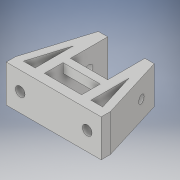
# Autodesk Inventor part: GT2_Holder
Saved by Autodesk Inventor 2018 (Build 220112000, 112)
## iProperties
Created: 2017-10-14
Part Number: GT2_Holder
Material: Generic
Document SubType Name: Modeling
Designer: Jurjen
Density: 1 g/cm^3
Appearance: Default
Author: Jurjen
Autodesk Inventor part; units mm, degrees
ref_plane "YZ Plane" through (0, 0, 0) normal (1, 0, 0) x (0, 1, 0)
ref_plane "XZ Plane" through (0, 0, 0) normal (0, 1, 0) x (-1, 0, 0)
ref_plane "XY Plane" through (0, 0, 0) normal (0, 0, 1) x (1, 0, 0)
sketch "Sketch1" plane through (0, 0, 0) normal (0, 0, 1) x (1, 0, 0)
  line L0 (-25.5, 10) -> (25.5, 10)
  line L1 (25.5, 10) -> (25.5, -10)
  line L2 (25.5, -10) -> (-25.5, -10)
  line L3 (-25.5, -10) -> (-25.5, 10)
  point P0 (0, 0)
  point P1 (0, 10)
  point P2 (25.5, 0)
  dimension "d0" = 51
  dimension "d1" = 20
  constraints: 8 end point, 2 midpoint, 2 parallel, 1 horizontal, 1 horizontal alignment, 1 perpendicular, 1 vertical alignment
  measures "d0" distance between parallel lines of L1 L3
  measures "d1" distance between parallel lines of L2 L0
extrude "Extrusion1" add sketch "Sketch1" along normal blind 5
sketch "Sketch2" plane through (-25.5, -10, 0) normal (0, -1, 0) x (1, 0, 0)
  line L0 (0, 0) -> (51, 0) projected
  line L1 (10.5, 0) -> (10.5, -34)
  line L2 (10.5, -34) -> (15.5, -34)
  line L3 (15.5, -34) -> (15.5, 0)
  line L4 (35.5, 0) -> (35.5, -34)
  line L5 (35.5, -34) -> (40.5, -34)
  line L6 (40.5, -34) -> (40.5, 0)
  line L7 (15.5, -34) -> (35.5, -34) construction
  line L8 (0, 0) -> (10.5, -34)
  line L9 (4.1864, 0) -> (10.5, -20.444)
  line L10 (51, 0) -> (40.5, -34)
  line L11 (40.5, -20.444) -> (46.8136, 0)
  point P0 (25.5, 0)
  point P1 (25.5, 0)
  point P2 (25.5, -34)
  dimension "d4" = 20
  dimension "d5" = 5
  dimension "d6" = 5
  dimension "d7" = 34
  dimension "d8" = 4
  dimension "d9" = 4
  constraints: 22 end point, 4 point on line, 3 parallel, 3 perpendicular, 2 horizontal, 1 midpoint, 1 vertical alignment, 8 other
  measures "d4" distance between parallel lines of L4 L3
  measures "d5" distance between parallel lines of L4 L6
  measures "d6" distance between parallel lines of L1 L3
  measures "d7" distance of the line from the sketch origin of L5
  measures "d8" distance between parallel lines of L9 L8
  measures "d9" distance between parallel lines of L10 L11
extrude "Extrusion2" add sketch "Sketch2" against normal up to surface (20 mm away) contours L0 L6 L5 L4 | L0 L9 L1 L8 | L1 L0 L3 L2 | L0 L10 L6 L11
sketch "Sketch3" plane through (10, -10, -34) normal (-1, 0, 0) x (0, 0, 1)
  circle A0 centre (10, 10) radius 2.1
  line L0 (0, 0) -> (0, 20) projected
  point P0 (34, 10)
  point P1 (0, 10)
  dimension "d12" = 4.2
  dimension "d13" = 10
  constraints: 1 centre point, 1 horizontal alignment, 1 midpoint
  measures "d12" diameter of A0
  measures "d13" distance from line of L0 A0.centre
extrude "Extrusion3" cut sketch "Sketch3" along normal blind 40 and the other way blind 40
sketch "Sketch4" plane through (-25.5, 10, 5) normal (0, 1, 0) x (1, 0, 0)
  line L0 (35.5, 15) -> (15.5, 15)
  line L1 (15.5, 15) -> (15.5, 19)
  line L2 (15.5, 19) -> (35.5, 19)
  line L3 (35.5, 19) -> (35.5, 15)
  line L4 (10.5, 39) -> (15.5, 39) projected
  point P0 (25.5, 5)
  point P1 (35.5, 5)
  point P2 (15.5, 5)
  dimension "d18" = 20
  dimension "d19" = 4
  constraints: 8 end point, 2 parallel, 2 vertical alignment, 1 horizontal, 1 perpendicular
  measures "d18" distance between parallel lines of L4 L2
  measures "d19" distance between parallel lines of L2 L0
extrude "Extrusion4" add sketch "Sketch4" against normal blind 5
sketch "Sketch6" plane through (0, 0, 5) normal (0, 0, 1) x (1, 0, 0)
  circle A0 centre (18, 0) radius 2.6
  circle A1 centre (-18, 0) radius 2.6
  point P0 (0, 0)
  dimension "d25" = 5.2
  dimension "d26" = 18
  dimension "d27" = 18
  constraints: 2 centre point, 2 horizontal alignment, 1 equal radius
  measures "d25" diameter of A1
  measures "d26" distance of A1.centre point (0, 0)
  measures "d27" distance of point (0, 0) A0.centre
extrude "Extrusion6" cut sketch "Sketch6" against normal blind 5
body "Solid1"
